ParaParamSample (Autodesk Fusion 360 design; units mm, degrees)
Autodesk Fusion 360 part; units mm, degrees
cylinder "CylinderPrimitive1" add diameter 25.4 height 25.4 placed x (1, 0, 0) y (0, 1, 0) z (0, 0, 1) at (0, 0, 0)
equation "Diameter = 1 in"
equation "Height = 1 in"
equation "d10 = Height"
equation "d11 = Diameter"
named bodies: "Body with Height and Diameter parameters"
